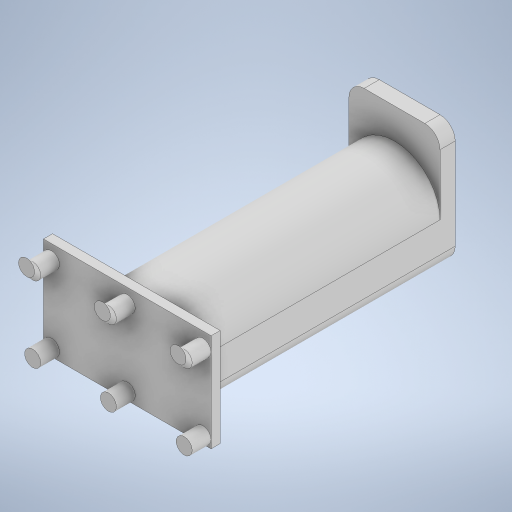
# Autodesk Inventor part: InvPegstr
Saved by Autodesk Inventor 2024 (Build 280153000, 153)
## iProperties
Created: 2024-12-11
Part Number: InvPegstr
Material: Типовые
Document SubType Name: Modeling
Designer: Admin
Density: 1 g/cm^3
Appearance: По умолчанию
Author: Admin
Autodesk Inventor part; units mm, degrees
ref_plane "YZ Plane" through (0, 0, 0) normal (1, 0, 0) x (0, 1, 0)
ref_plane "XZ Plane" through (0, 0, 0) normal (0, 1, 0) x (-1, 0, 0)
ref_plane "XY Plane" through (0, 0, 0) normal (0, 0, 1) x (1, 0, 0)
sketch "Эскиз1" plane through (0, 0, 0) normal (0, 0, 1) x (1, 0, 0)
  line L0 (-27.6, 16.125) -> (27.6, 16.125)
  line L1 (27.6, 16.125) -> (27.6, -16.125)
  line L2 (27.6, -16.125) -> (-27.6, -16.125)
  line L3 (-27.6, -16.125) -> (-27.6, 16.125)
  line L4 (-27.6, 16.125) -> (27.6, -16.125) construction
  line L5 (27.6, 16.125) -> (-27.6, -16.125) construction
  point P0 (0, 0)
  dimension "d2" = 55.2
  dimension "d3" = 32.25
  constraints: 12 end point, 2 midpoint, 2 parallel, 1 horizontal, 1 perpendicular
  measures "d2" distance of L0.start L0.end
  measures "d3" distance of L2.end L0.start
extrude "Выдавливание1" add sketch "Эскиз1" along normal blind 1.85
sketch "Эскиз2" plane through (0, 0, 1.85) normal (0, 0, 1) x (1, 0, 0)
  line L0 (-27.6, 16.125) -> (-27.6, -16.125) construction
  circle A0 centre (-24.95, 11.475) radius 2.65
  line L1 (0, 0) -> (0, 16.125) construction
  line L2 (27.6, 16.125) -> (-27.6, 16.125) construction
  line L3 (0, 0) -> (-27.6, 0) construction
  dimension "d4" = 5.3
  dimension "d51" = 2
  constraints: 4 end point, 2 midpoint, 1 centre point, 1 tangent
  measures "d4" diameter of A0
  measures "d51" distance edge to line of A0 L2
extrude "Выдавливание2" add sketch "Эскиз2" along normal blind 6.2
pattern_linear "Прямоуг.массив1" count 3 spacing 24.95 along (1, 0, 0) count 2 spacing 24.95 along (0, -1, 0) of "Выдавливание2"
sketch "Эскиз3" plane through (-27.6, 16.125, 0) normal (0, -1, 0) x (1, 0, 0)
  line L0 (47.5, -16.8) -> (7.7, -16.8)
  line L1 (7.7, -16.8) -> (7.7, 0)
  line L2 (7.7, 0) -> (47.5, 0)
  line L3 (47.5, 0) -> (47.5, -16.8)
  line L4 (0, 0) -> (55.2, 0) projected
  point P0 (27.6, 0)
  point P1 (27.6, 0)
  point P2 (27.6, 0)
  dimension "d46" = 39.8
  dimension "d47" = 16.8
  constraints: 8 end point, 3 midpoint, 2 coincident, 2 parallel, 1 horizontal, 1 perpendicular
  measures "d46" distance of L0.start L0.end
  measures "d47" distance of L0.end L1.end
extrude "Выдавливание3" add sketch "Эскиз3" along normal blind 31.1875
sketch "Эскиз4" plane through (-27.6, 16.125, 1.85) normal (0, 1, 0) x (1, 0, 0)
  line L0 (45.1, 6.25) -> (10.1, 6.25)
  line L1 (10.1, 6.25) -> (10.1, 16.25)
  line L2 (10.1, 16.25) -> (45.1, 16.25)
  line L3 (45.1, 16.25) -> (45.1, 6.25)
  line L4 (7.7, 18.65) -> (47.5, 18.65) projected
  line L5 (47.5, 18.65) -> (47.5, 1.85) projected
  point P0 (47.5, 1.85)
  point P1 (32.525, 1.85)
  dimension "d27" = 35
  dimension "d31" = 10
  dimension "d55" = 2.4
  dimension "d56" = 2.4
  constraints: 8 end point, 2 perpendicular, 1 other
  measures "d27" distance of L1.end L2.end
  measures "d31" distance of L0.end L1.end
  measures "d55" distance between parallel lines of L4 L2
extrude "Выдавливание4" cut sketch "Эскиз4" against normal blind 29.1875
fillet "Сопряжение1" radius 2 4 edges at (-17.5, 1.5312, -4.4) (-17.5, 1.5312, -14.4) (17.5, 1.5312, -4.4) (17.5, 1.5312, -14.4)
pattern_of_one "Прямоуг.массив2"
fillet "Сопряжение2" radius 2 2 edges at (19.9, 0.5313, -16.8) (-19.9, 0.5312, -16.8)
ref_plane "РабПлоскость1" through (-24.95, 11.475, 10.05) normal (0, 0, 1) x (1, 0, 0)
sketch "Эскиз7" plane through (-24.95, 11.475, 10.05) normal (0, 0, 1) x (1, 0, 0)
  circle A0 centre (0, 0) radius 2.65 construction
  circle A1 centre (0, 2) radius 2.65
  point P0 (24.95, -11.475)
  dimension "d60" = 5.3
  dimension "d61" = 2
  constraints: 1 centre point, 1 vertical alignment
  measures "d60" diameter of A1
  measures "d61" distance of A0.centre A1.centre
loft "Лофт1" add profiles "Эскиз7" section 1 edges at (-27.6, 11.475, 8.05)
pattern_linear "Прямоуг.массив3" count 3 spacing 24.95 along (1, 0, 0) of "Лофт1"
delete faces "Удаление грани1" heal yes whole lump no faces at (5.9667, -15.0625, -5.6)
move faces "Перенос1" translate (0, 0, -1.15) faces at (-9.2, -5.375, 0)
sketch "Эскиз10" plane through (27.6, -16.125, -1.15) normal (0, 0, -1) x (-1, 0, 0)
  circle A0 centre (27.6, 15) radius 15
  line L0 (12.6, 15) -> (42.6, 15)
  line L1 (42.6, 15) -> (42.6, 0)
  line L2 (42.6, 0) -> (12.6, 0)
  line L3 (12.6, 0) -> (12.6, 15)
  line L4 (55.2, 0) -> (0, 0) projected
  line L5 (0, 32.25) -> (55.2, 32.25) projected
  point P0 (27.6, 0)
  point P1 (27.6, 32.25)
  point P2 (27.6, 0)
  point P3 (42.6, 15)
  dimension "d70" = 30
  constraints: 8 end point, 3 midpoint, 2 coincident, 2 horizontal, 2 parallel, 2 vertical alignment, 1 collinear, 1 perpendicular, 1 vertical, 3 other
extrude "Выдавливание6" add sketch "Эскиз10" along normal blind 85
sketch "Эскиз11" plane through (0, -1.125, -86.15) normal (0, 0, -1) x (1, 0, 0)
  circle A0 centre (0, -1.125) radius 20
  line L0 (20, -1.125) -> (-20, -1.125)
  line L1 (-20, -1.125) -> (-20, 15)
  line L2 (-20, 15) -> (20, 15)
  line L3 (20, 15) -> (20, -1.125)
  line L4 (15, 15) -> (-15, 15) projected
  line L5 (20, -1.125) -> (-20, -1.125)
  line L6 (-20, -1.125) -> (-20, -21.125)
  line L7 (-20, -21.125) -> (20, -21.125)
  line L8 (20, -21.125) -> (20, -1.125)
  line L9 (20, -21.125) -> (-20, -21.125)
  line L10 (-20, -21.125) -> (-20, -25)
  line L11 (-20, -25) -> (20, -25)
  line L12 (20, -25) -> (20, -21.125)
  point P0 (0, -21.125)
  dimension "d76" = 40
  dimension "d80" = 40
  constraints: 24 end point, 6 parallel, 4 horizontal, 3 perpendicular, 2 vertical, 1 coincident, 1 collinear, 3 other
  measures "d80" distance between parallel lines of L2 L11
extrude "Выдавливание7" add sketch "Эскиз11" along normal blind 5 contours L0 A0 L2 | L8 L7 A0 | A0 L0 | A0 L2 L3 | L7 L6 A0 | L7 L12 L11 L10 | L1 L2 A0
fillet "Сопряжение3" radius 5 2 edges at (15, -16.125, -43.65) (-15, -16.125, -43.65)
move faces "Перенос2" translate (-5, 0, 0) faces at (20, 10.5417, -89.4833)
move faces "Перенос3" translate (5, 0, 0) faces at (-20, -2.7917, -89.4833)
delete faces "Удаление грани2" heal yes whole lump no faces at (-14.0089, -15.1339, -86.15) (14.0089, -15.1339, -86.15)
fillet "Сопряжение4" radius 5 2 edges at (-15, 23.875, -88.65) (15, 23.875, -88.65)
equation "\"d2\" = iTotalWidth"
equation "\"d3\" = iTotalHeight"
equation "\"iTotalWidth\" = 55.2"
equation "\"iTotalHeight\" = 32.25"
equation "\"iTotalHolderXSize\" = 39.8"
equation "\"iTotalHolderYSize\" = 16.8"
